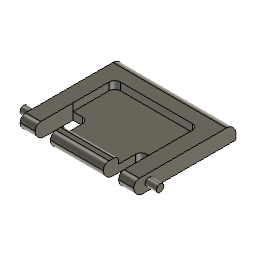
kick stand (Autodesk Fusion 360 design; units mm, degrees)
Autodesk Fusion 360 part; units mm, degrees
note: some values were not read from the file. Set by a fixed rule: which sketch regions a step uses.
sketch "Sketch1" plane through (0, 0, 0) normal (0, 0, 1) x (1, 0, 0)
  line L0 (0, 0) -> (2, 0)
  line L1 (2, 0) -> (6, 0)
  line L2 (6, 0) -> (6, 10)
  line L3 (6, 10) -> (10, 10)
  line L4 (10, 10) -> (10, 0)
  line L5 (10, 0) -> (24, 0)
  line L6 (24, 0) -> (24, 10)
  line L7 (24, 10) -> (28, 10)
  line L8 (28, 10) -> (28, 0)
  line L9 (28, 0) -> (32, 0)
  line L10 (32, 0) -> (34, 0)
  line L11 (34, 0) -> (34, 2)
  line L12 (34, 2) -> (32, 2)
  line L13 (32, 2) -> (32, 27)
  line L14 (0, 0) -> (0, 2)
  line L15 (0, 2) -> (2, 2)
  line L16 (2, 2) -> (2, 27)
  line L17 (2, 27) -> (32, 27)
  line L18 (2, 2) -> (2, 0)
  line L19 (32, 2) -> (32, 0)
  dimension "d1" = 2
  dimension "d2" = 4
  dimension "d3" = 10
  dimension "d4" = 4
  dimension "d5" = 14
  dimension "d6" = 4
  dimension "d7" = 4
  dimension "d8" = 2
  dimension "d9" = 2
  dimension "d10" = 2
  dimension "d11" = 25
  dimension "d12" = 2
  dimension "d13" = 2
  dimension "d14" = 25
  dimension "d43" = 30
  constraint coincident L0.start L14.start
  constraint horizontal L0
  constraint parallel L0 L1
  constraint perpendicular L1 L2
  constraint perpendicular L2 L3
  constraint perpendicular L1 L4
  constraint perpendicular L4 L5
  constraint perpendicular L5 L6
  constraint perpendicular L6 L7
  constraint perpendicular L7 L8
  constraint perpendicular L8 L9
  constraint perpendicular L8 L10
  constraint perpendicular L10 L11
  constraint perpendicular L8 L12
  constraint perpendicular L12 L13
  constraint parallel L2 L14
  constraint perpendicular L2 L15
  constraint perpendicular L15 L16
  constraint perpendicular L13 L17
  measures "d1" distance of L0.start L0.end
  measures "d2" distance of L0.end L1.end
  measures "d3" distance of L1.end L2.end
  measures "d4" distance of L2.end L3.end
  measures "d5" distance of L4.end L5.end
  measures "d6" distance of L6.end L7.end
  measures "d7" distance of L8.end L9.end
  measures "d8" distance of L9.end L10.end
  measures "d9" distance of L10.end L11.end
  measures "d10" distance of L11.end L12.end
  measures "d11" distance of L12.end L13.end
  measures "d12" distance of L0.start L14.end
  measures "d13" distance of L14.end L15.end
  measures "d14" distance of L15.end L16.end
  measures "d43" distance of L13.end L16.end
extrude "Extrude1" add sketch "Sketch1" along normal blind 4 contours L1 L2 L3 L4 L5 L6 L7 L8 L9 L13 L16 L17 L18 L19
sketch "Sketch2" plane through (32, 0, 0) normal (1, 0, 0) x (0, 1, 0)
  line L0 (0, 0) -> (27, 0)
  line L1 (27, 0) -> (27, 4)
  line L2 (27, 4) -> (0, 4)
  line L3 (0, 4) -> (0, 0)
  circle A0 centre (4, 2) radius 1
  dimension "d17" = 2
  dimension "d56" = 2
  dimension "d57" = 4
  measures "d17" diameter of A0
  measures "d56" distance of L2 A0.centre
  measures "d57" distance of L3 A0.centre
sketch "Sketch3" plane through (32, 0, 0) normal (1, 0, 0) x (0, 1, 0)
  line L0 (0, 4) -> (0, 0)
  line L1 (0, 4) -> (0, 2)
  line L2 (0, 2) -> (4.8814, 2)
  point P0 (0, 4)
  constraint coincident P0 L0.start
  constraint midpoint L0 L1.end
  constraint perpendicular L1 L2
extrude "Extrude2" add sketch "Sketch2" along normal blind 3 contours A0
sketch "Sketch4" plane through (2, 0, 0) normal (-1, 0, 0) x (0, -1, 0)
  line L0 (-27, 0) -> (0, 0)
  line L1 (0, 0) -> (0, 4)
  line L2 (0, 4) -> (-27, 4)
  line L3 (-27, 4) -> (-27, 0)
  circle A0 centre (-4, 2) radius 1
  line L4 (0, 0) -> (0, 2)
  dimension "d20" = 2
  dimension "d54" = 2
  dimension "d55" = 4
  constraint coincident L0.end L1.start
  constraint midpoint L1 L4.end
  measures "d20" diameter of A0
  measures "d54" distance of L2 A0.centre
  measures "d55" distance of A0.centre L4
extrude "Extrude3" add sketch "Sketch4" along normal blind 3 contours A0
fillet "Fillet1" radius 2.5 1 edges at (17, 27, 4)
sketch "Sketch5" plane through (0, 0, 4) normal (0, 0, 1) x (-1, 0, 0)
  line L0 (-32, -24.5) -> (-2, -24.5)
  line L1 (-2, -24.5) -> (-2, 0)
  line L2 (-2, 0) -> (-6, 0)
  line L3 (-6, 0) -> (-6, -10)
  line L4 (-6, -10) -> (-10, -10)
  line L5 (-10, -10) -> (-10, 0)
  line L6 (-10, 0) -> (-24, 0)
  line L7 (-24, 0) -> (-24, -10)
  line L8 (-24, -10) -> (-28, -10)
  line L9 (-28, -10) -> (-28, 0)
  line L10 (-28, 0) -> (-32, 0)
  line L11 (-32, 0) -> (-32, -24.5)
  line L12 (-28, -6.2874) -> (-16.9, -6.2874)
  line L13 (-16.9, -6.2874) -> (-16.9, -24.5)
  line L14 (-16.9, -24.5) -> (-28, -24.5)
  line L15 (-28, -24.5) -> (-28, -6.2874)
  constraint horizontal L12
  constraint vertical L13
  constraint horizontal L14
  constraint vertical L15
  constraint coincident L0 L13.end
  constraint coincident L9 L12.start
extrude "Extrude4" cut sketch "Sketch5" against normal blind 2 contours L0 L7 L8 L12 L13 L14 L15
fillet "Fillet2" radius 1.5 1 edges at (17, 0, 4)
fillet "Fillet3" radius 1.5 1 edges at (4, 0, 4)
fillet "Fillet4" radius 1.5 1 edges at (30, 0, 4)
sketch "Sketch6" plane through (0, 0, 2) normal (0, 0, 1) x (-1, 0, 0)
  line L0 (-16.9, -6.2874) -> (-24, -6.2874)
  line L1 (-24, -6.2874) -> (-24, -10)
  line L2 (-24, -10) -> (-28, -10)
  line L3 (-28, -10) -> (-28, -24.5)
  line L4 (-28, -24.5) -> (-16.9, -24.5)
  line L5 (-16.9, -24.5) -> (-16.9, -6.2874)
  line L6 (-28, -24.5) -> (-3.7012, -24.5)
  line L7 (-3.7012, -24.5) -> (-3.7012, -19.6935)
  line L8 (-28, -19.6935) -> (-28, -24.5)
  constraint horizontal L6
  constraint vertical L7
  constraint vertical L8
  constraint coincident L3.end L4.start
extrude "Extrude6" add sketch "Sketch6" along normal blind 2
fillet "Fillet9" radius 1.5 2 edges at (10, 10, 2) (24, 10, 2)
extrude "Extrude5" add sketch "Sketch6" along normal blind 2
sketch "Sketch7" plane through (0, 0, 4) normal (0, 0, 1) x (-1, 0, 0)
  line L0 (-28, -10) -> (-28, -1.5)
  line L1 (-28, -1.5) -> (-32, -1.5)
  line L2 (-32, -1.5) -> (-32, -24.5)
  line L3 (-32, -24.5) -> (-2, -24.5)
  line L4 (-2, -24.5) -> (-2, -1.5)
  line L5 (-2, -1.5) -> (-6, -1.5)
  line L6 (-6, -1.5) -> (-6, -10)
  line L7 (-6, -10) -> (-8.5, -10)
  arc A0 (-10, -8.5) -> (-8.5, -10) centre (-8.5, -8.5) ccw
  line L8 (-10, -8.5) -> (-10, -1.5)
  line L9 (-10, -1.5) -> (-24, -1.5)
  line L10 (-24, -1.5) -> (-24, -8.5)
  arc A1 (-25.5, -10) -> (-24, -8.5) centre (-25.5, -8.5) ccw
  line L11 (-25.5, -10) -> (-28, -10)
  line L12 (-24, -4) -> (-10, -4)
  line L13 (-28, -10) -> (-28, -22)
  line L14 (-28, -22) -> (-6, -22)
  line L15 (-6, -22) -> (-6, -10)
  constraint coincident L10 L12.start
  constraint coincident L8 L12.end
  constraint perpendicular L8 L12
  constraint coincident L0.start L11.end
  constraint perpendicular L11 L13
  constraint perpendicular L13 L14
  constraint coincident L6.end L7.start
extrude "Extrude7" cut sketch "Sketch7" against normal blind 2 contours L7 A0 L8 L10 A1 L11 L12 L13 L14 L15
extrude "Extrude8" add 1 faces at (20.6667, 22, 3.3333) along direction (0, -1, 0) blind 1
fillet "Fillet10" radius 1.5 2 edges at (6, 21, 3) (28, 21, 3)
fillet "Fillet11" radius 2.5 3 edges at (17, 0, 0) (4, 0, 0) (30, 0, 0)
fillet "Fillet12" radius 1.25 1 edges at (17, 4, 4)
